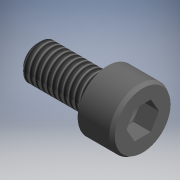
# Autodesk Inventor part: CBM5-10
Saved by Autodesk Inventor 2017.3 (Build 213256000, 256)
## iProperties
Part Number: CBM5-10
Material: Generic
Catalog Web Link: www.cadenas.de
Description: CBM-Hex Socket Head Cap Screws - Bright Chromate Plating
Vendor: MISUMI
Document SubType Name: Modeling
Designer: partserver
Manufacturer: MISUMI
Mass: 0.437085 g
Surface Area: 4.2861 cm^2
Volume: 0.437085 cm^3
Density: 1 g/cm^3
Appearance: PSOLRGB-128-128-128
Category: PARTsolutions
Company: MISUMI
Title: CBM5-10
Author: Cadenas PARTsolutions
Comments: Hex Socket Head Cap Screws - Bright Chromate Plating
PSOL_IDENT_0: {$CADENAS_DATA\23d-libs\misumi\metric\27_screws_nuts\cbm.prj},153 {VTYP=3D},{NB=CBM5-10},{LINA=CBM5-
PSOL_IDENT_1: 10},{NN=CBM},{DATE=07.06.2021 12:24:55},{GEOMDATE=24.03.2015 11:44:00},{VERSION=},{LINEID=40},{WBVAR=
PSOL_IDENT_2: L},{WBNUMERIC=L}  {NB=CBM5-10},{LINA=CBM5-10},{KT=DUMMY},{PN=CBM5-10},{TYPE=CBM},{M=5},{M1=5},{L=10}
PSOL_IDENT_3: ,{LALG=6,8,10,12,14,15,18,20,22,25,30,35,40,45,50},{LL=Studs - Fully Threaded},{A=8.5},{E=5},{B=4.0}
PSOL_IDENT_4: ,{LL3D=9.8},{TT3D=2.5},{R3D=0.200},{C3D=0.5},{A3D=-60}
NB: CBM5-10
NN: CBM
NT: Hex Socket Head Cap Screws - Bright Chromate Plating
NBSYN: $PN.
LINA: CBM5-10
CATALOG: Misumi
PN: CBM5-10
M: 5
L: 10
LL: Studs - Fully Threaded
A: 8.5
E: 5
B: 4
SUPPLIER: MISUMI
ARTICLENO: CBM5-10
BOMINFO: CBM5-10
CREATOR: CADENAS GmbH
Autodesk Inventor part; units mm, degrees
sketch "Sketch_8" plane through (0, 0, 0) normal (0, 0, 1) x (1, 0, 0)
  line L0 (10, 0) -> (-5, 0)
  line L1 (-5, 0) -> (-5, 3.9613)
  line L2 (-5, 3.9613) -> (-4.5, 4.25)
  line L3 (-4.5, 4.25) -> (0, 4.25)
  line L4 (0, 4.25) -> (0, 2.7)
  arc A0 (0, 2.7) -> (0.2, 2.5) centre (0.2, 2.7) ccw
  line L5 (0.2, 2.5) -> (9.5095, 2.5)
  line L6 (9.5095, 2.5) -> (10, 2.0095)
  line L7 (10, 2.0095) -> (10, 0)
  line L8 (10, 0) -> (-5, 0)
  constraints: 18 end point, 2 point on circle, 1 centre point
revolve "Revolution1" add sketch "Sketch_8" angle 360 about axis through (10, 0, 0) along (1, 0, 0)
thread "Thread1" size "M5x0.8" class "6g" standard "ISO Metric profile" full length
sketch "Sketch2" plane through (-5, 0, 0) normal (-1, 0, 0) x (0, 0, 1)
  point P0 (0, 0)
hole "Hole1" at (-5, 0, 0) direction (1, 0, 0) diameter 4 depth 2.5 tip angle 120
sketch "Sketch_3" plane through (-5, 0, 0) normal (1, 0, 0) x (0, 0, -1)
  line L0 (-2, -1.1547) -> (0, -2.3094)
  line L1 (0, -2.3094) -> (2, -1.1547)
  line L2 (2, -1.1547) -> (2, 1.1547)
  line L3 (2, 1.1547) -> (0, 2.3094)
  line L4 (0, 2.3094) -> (-2, 1.1547)
  line L5 (-2, 1.1547) -> (-2, -1.1547)
  constraints: 12 end point
extrude "Extrusion1" cut sketch "Sketch_3" along normal blind 2.5
ref_plane "bolt_XY" through (0, 0, 0) normal (1, 0, 0) x (0, 0, -1)
ref_plane "bolt_YZ" through (0, 0, 0) normal (0, 0, -1) x (0, 1, 0)
ref_plane "bolt_ZX" through (0, 0, 0) normal (0, 1, 0) x (1, 0, 0)
ref_plane "nut_XY" through (10, 0, 0) normal (1, 0, 0) x (0, 0, -1)
ref_plane "nut_YZ" through (10, 0, 0) normal (0, 0, -1) x (0, 1, 0)
ref_plane "nut_ZX" through (10, 0, 0) normal (0, 1, 0) x (1, 0, 0)
body "Solid1"
